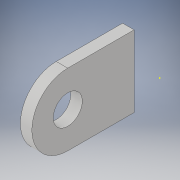
# Autodesk Inventor part: Part11
Saved by Autodesk Inventor 2019 (Build 230136000, 136)
## iProperties
Created: 2021-08-30
Part Number: Part11
Material: 一般
Document SubType Name: Sheet Metal
Designer: yuta
Density: 1 g/cm^3
Sheet Metal Rule: Default_mm
Appearance: 既定
Author: yuta
Autodesk Inventor part; units mm, degrees
ref_plane "YZ Plane" through (0, 0, 0) normal (1, 0, 0) x (0, 1, 0)
ref_plane "XZ Plane" through (0, 0, 0) normal (0, 1, 0) x (-1, 0, 0)
ref_plane "XY Plane" through (0, 0, 0) normal (0, 0, 1) x (1, 0, 0)
sketch "スケッチ1" plane through (0, 0, 0) normal (1, 0, 0) x (0, 1, 0)
  line L0 (6.1647, 10.3826) -> (-1.9353, 10.3826)
  line L1 (-1.9353, 10.3826) -> (-1.9353, 2.8826)
  line L2 (-1.9353, 2.8826) -> (6.1647, 2.8826)
  line L3 (6.1647, 2.8826) -> (6.1647, 10.3826)
  arc A0 (6.1647, 10.3826) -> (-1.9353, 10.3826) centre (2.1147, 10.3826) ccw
  circle A1 centre (2.1147, 10.3826) radius 1.64
  point P0 (0, 0)
  dimension "d0" = 8.1
  dimension "d1" = 7.5
  dimension "d2" = 3.28
  constraints: 8 end point, 2 centre point, 2 parallel, 2 point on circle, 2 tangent, 1 coincident, 1 horizontal, 1 perpendicular
  measures "d0" distance of L2.end L1.end
  measures "d1" distance of L1.end L0.end
  measures "d2" diameter of A1
extrude "押し出し1" add sketch "スケッチ1" along normal blind 1.3
sketch "スケッチ2" plane through (1.3, 0, 0) normal (1, 0, 0) x (0, 0, -1)
  point P0 (0, 0)
sketch "スケッチ3" plane through (1.3, 0, 0) normal (1, 0, 0) x (0, 0, -1)
  arc A0 (-10.3826, 6.1647) -> (-10.3826, -1.9353) centre (-10.3826, 2.1147) ccw projected
  circle A1 centre (-10.3826, 2.1147) radius 1.64
  point P0 (0, 0)
  dimension "d6" = 3.28
  constraints: 1 centre point, 1 coincident
  measures "d6" diameter of A1
hole "穴1" at (1.3, 2.1147, 10.3826) direction (-1, 0, 0) diameter 3.28 depth 1.3
equation "\"BendRadius\" = Thickness"
equation "\"BendReliefWidth\" = Thickness"
equation "\"BendReliefDepth\" = 0.5 * Thickness"
equation "\"CornerReliefSize\" = 4 * Thickness"
equation "\"MinimumRemnant\" = 2 * Thickness"
equation "\"TransitionRadius\" = BendRadius"
equation "\"JacobiRadiusSize\" = BendRadius"
equation "\"GapSize\" = Thickness"
equation "\"Thickness\" = 0.5"
